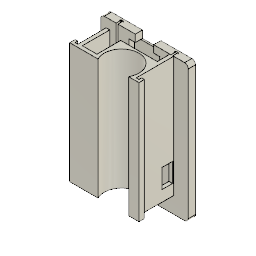
Battery Case v1 (Autodesk Fusion 360 design; units mm, degrees)
Autodesk Fusion 360 part; units mm, degrees
note: some values were not read from the file. Chosen so that the rebuilt part matches the saved one: which face or edge a step refers to; where a step starts. Set by a fixed rule: which sketch regions a step uses.
sketch "Bottom" plane through (0, 0, 0) normal (0, 1, 0) x (1, 0, 0) in component "Battery"
  line L0 (32.7362, 0) -> (32.7362, -7)
  line L1 (32.7362, -7) -> (12.7362, -7)
  line L2 (12.7362, -7) -> (12.7362, -20)
  line L3 (4.7362, 0) -> (4.7362, -20)
  line L4 (4.7362, -20) -> (12.7362, -20)
  line L5 (2.7362, 0) -> (2.7362, -20.5)
  line L6 (-0.2638, -22) -> (-0.2638, -19)
  line L7 (-0.2638, -19) -> (1.2362, -19)
  line L8 (1.2362, -19) -> (1.2362, -20.5)
  line L9 (1.2362, -20.5) -> (2.7362, -20.5)
  line L10 (37.7362, -22) -> (37.7362, -19)
  line L11 (37.7362, -19) -> (36.2362, -19)
  line L12 (36.2362, -19) -> (36.2362, -20.5)
  line L13 (36.2362, -20.5) -> (34.7362, -20.5)
  line L14 (-0.2638, -22) -> (15.3696, -22)
  line L15 (32.1028, -22) -> (37.7362, -22)
  line L16 (34.7362, 0) -> (34.7362, -20.5)
  line L17 (0, 0) -> (2.7362, 0) construction
  line L18 (4.2362, 0) -> (4.2362, 2.4992)
  line L19 (4.3455, 3) -> (4.8463, 2.4992)
  line L20 (3.2362, 2.4992) -> (3.2362, 0)
  line L21 (3.127, 3) -> (2.6261, 2.4992)
  line L22 (4.2362, 2.4992) -> (4.8463, 2.4992)
  line L23 (2.6261, 2.4992) -> (3.2362, 2.4992)
  line L24 (3.7361, 3) -> (3.7362, 0) construction
  line L25 (2.7362, 0) -> (4.7362, 0)
  line L26 (3.127, 3) -> (4.3455, 3)
  line L27 (32.6219, 2.4973) -> (33.232, 2.4983)
  line L28 (33.1209, 3) -> (32.6219, 2.4973)
  line L29 (33.1209, 3) -> (34.3394, 3)
  line L30 (33.7361, 3) -> (33.7362, 0) construction
  line L31 (34.232, 2.5) -> (34.8421, 2.501)
  line L32 (34.3394, 3) -> (34.8421, 2.501)
  line L33 (33.232, 2.4983) -> (33.2362, 0)
  line L34 (34.2362, 0) -> (34.232, 2.5)
  line L35 (32.7362, 0) -> (34.7362, 0)
  line L36 (15.3696, -22) -> (32.1028, -22) construction
  line L37 (23.7362, -22) -> (23.7362, -8) construction
  arc A0 (32.1028, -22) -> (15.3696, -22) centre (23.7362, -17.5) ccw
  dimension "d8" = 32
  dimension "d43" = 0
  dimension "d44" = 0
  dimension "d45" = 0
  dimension "d46" = 0
  dimension "d65" = 1.5
  dimension "d66" = 1.5
  dimension "d68" = 1.5
  dimension "d69" = 1.5
  dimension "d70" = 3
  dimension "d71" = 3
  dimension "d72" = 15.6334
  dimension "d73" = 5.6334
  dimension "d74" = 20.5
  dimension "d75" = 20
  dimension "d76" = 8
  dimension "d77" = 1.5
  dimension "d79" = 20
  dimension "d80" = 13
  dimension "d81" = 7
  dimension "d82" = 2
  dimension "d83" = 20.5
  dimension "d84" = 1.5
  dimension "d85" = 2.7362
  dimension "d94" = 1
  dimension "d98" = 0.6101
  dimension "d99" = 0.7083
  dimension "d100" = 1.2185
  dimension "d101" = 0.5
  dimension "d102" = 0.6101
  dimension "d103" = 0.7083
  dimension "d105" = 2
  dimension "d106" = 3
  dimension "d107" = 1
  dimension "d108" = 0.6101
  dimension "d109" = 0.7083
  dimension "d110" = 1.2185
  dimension "d112" = 0.6101
  dimension "d113" = 0.7083
  dimension "d116" = 0.5
  dimension "d117" = 3
  dimension "d118" = 2.5
  dimension "d132" = 19
  measures "d8" distance of L16.start L5.start
  measures "d65" distance of L6.end L7.end
  measures "d66" distance of L7.end L8.end
  measures "d68" distance of L11.end L12.end
  measures "d69" distance of L10.end L11.end
  measures "d70" distance of L6.start L6.end
  measures "d71" distance of L10.start L10.end
  measures "d72" distance of L14.end L6.start
  measures "d73" distance of L15.start L10.start
  measures "d74" distance of L5.start L5.end
  measures "d75" distance of L3.start L3.end
  measures "d76" distance of L3.end L2.end
  measures "d77" distance of L8.end L5.end
  measures "d79" distance of L0.end L1.end
  measures "d80" distance of L1.end L2.end
  measures "d81" distance of L0.start L0.end
  measures "d82" distance of L16.start L0.start
  measures "d83" distance of L16.start L13.end
  measures "d84" distance of L12.end L13.end
  measures "d85" distance of L5.start L17.start
  measures "d94" distance of L20.end L18.start
  measures "d98" distance of L19.end L18.end
  measures "d99" distance of L19.end L19.start
  measures "d100" distance of L21.start L19.start
  measures "d101" distance of L5.start L20
  measures "d102" distance of L21.end L20.start
  measures "d103" distance of L21.end L21.start
  measures "d105" distance of L3.start L5.start
  measures "d106" distance of L25 L26
  measures "d107" distance of L33.end L34.start
  measures "d108" distance of L31.start L31.end
  measures "d109" distance of L31.end L29.end
  measures "d110" distance of L28.start L29.end
  measures "d112" distance of L27.start L27.end
  measures "d113" distance of L27.start L28.start
  measures "d116" distance of L0.start L33
  measures "d117" distance of L29 L35
  measures "d118" distance of L31.start L34.start
  measures "d132" diameter of A0
extrude "Extrude1" add sketch "Bottom" along normal blind 66 contours L0 L1 L2 L3 L4 L5 L6 L7 L8 L9 L10 L11 L12 L13 L14 L15 L16 L25 L35 A0 makes body 1 in component "Battery"
sketch "Side" plane through (2.7362, 0, 0) normal (-1, 0, 0) x (0, 0, 1) in component "Battery"
  line L0 (0, 0) -> (20.5, 0)
  line L1 (20.5, 66) -> (0, 66)
  line L2 (0, 66) -> (5, 66)
  line L3 (5, 66) -> (5, 56)
  line L4 (5, 56) -> (0, 56)
  line L5 (0, 0) -> (5, 0)
  line L6 (5, 0) -> (5, 10)
  line L7 (5, 10) -> (0, 10)
  line L8 (20.5, 0) -> (20.5, 66)
  line L9 (0, 66) -> (0, 0)
  dimension "d86" = 10
  dimension "d87" = 5
  dimension "d88" = 10
  dimension "d89" = 5
  measures "d86" distance of L5.end L6.end
  measures "d87" distance of L6.end L7.end
  measures "d88" distance of L2.end L3.end
  measures "d89" distance of L3.end L4.end
extrude "Extrude2" cut sketch "Side" against normal blind 2 contours L0 L5 L6 L7 L9 | L1 L2 L3 L4 L9 bodies 1 in component "Battery"
sketch "Right Side" plane through (34.7362, 0, 0) normal (1, 0, 0) x (0, 0, -1) in component "Battery"
  line L0 (-22, 0) -> (0, 0)
  line L1 (0, 0) -> (0, 66)
  line L2 (0, 66) -> (-22, 66)
  line L3 (-22, 66) -> (-22, 0)
  line L4 (-0.6, 6) -> (-0.6, 16.5)
  line L5 (-6.4, 16.5) -> (-6.4, 6)
  line L6 (-0.6, 16.5) -> (-6.4, 16.5)
  line L7 (-6.4, 16.5) -> (-0.6, 16.5)
  line L8 (-0.6, 16.5) -> (-0.6, 6)
  line L9 (-0.6, 6) -> (-6.4, 6)
  line L10 (-6.4, 6) -> (-6.4, 16.5)
  line L11 (-20.5, 0) -> (0, 0)
  line L12 (0, 66) -> (-20.5, 66)
  line L13 (-20.5, 66) -> (-20.5, 0)
  line L14 (-0.6, 6) -> (0, 6) construction
  line L15 (0, 0) -> (0, 66)
  dimension "d14" = 10.5
  dimension "d90" = 6
  dimension "d91" = 0.6
  dimension "d92" = 5.8
  measures "d14" distance of L5.start L5.end
  measures "d90" distance of L0.end L14.end
  measures "d91" distance of L4.start L14.end
  measures "d92" distance of L4.start L5.end
extrude "Extrude3" cut sketch "Right Side" against normal blind 3 contours L4 L5 L6 L7 L8 L9 L10 bodies 1 in component "Battery"
extrude "Extrude9" add sketch "Bottom" against normal blind 40 from surface at 56 contours L18 L19 L20 L21 L22 L23 L25 L26 bodies 1 in component "Battery"
extrude "Extrude11" add sketch "Bottom" against normal blind 50 from surface at 66 contours L27 L28 L29 L31 L32 L33 L34 L35 bodies 1 in component "Battery"
extrude "Extrude10" cut sketch "Bottom" along normal blind 20 from surface at 26 contours L18 L19 L20 L21 L22 L23 L25 L26 bodies 1 in component "Battery"
extrude "Extrude12" cut sketch "Bottom" against normal blind 30 from surface at 56 contours L27 L28 L29 L31 L32 L33 L34 L35 bodies 1 in component "Battery"
sketch "Bottom (2)" plane through (0, 0, 0) normal (0, 1, 0) x (1, 0, 0) in component "Charger"
  line L0 (24, -2) -> (24, -73)
  line L1 (22, -75) -> (-22, -75)
  line L2 (-24, -73) -> (-24, -2)
  arc A0 (-22, 0) -> (-24, -2) centre (-22, -2) ccw
  arc A1 (24, -2) -> (22, 0) centre (22, -2) ccw
  arc A2 (22, -75) -> (24, -73) centre (22, -73) ccw
  arc A3 (-24, -73) -> (-22, -75) centre (-22, -73) ccw
  line L3 (5, 0) -> (5, -4)
  line L4 (5, -4) -> (-5, -4)
  line L5 (-5, -4) -> (-5, 0)
  line L6 (15.5, 0) -> (15.5, -50)
  line L7 (-15.5, -50) -> (-15.5, 0)
  line L8 (-15.5, 0) -> (-14.5, 0)
  line L9 (-14.5, 0) -> (-14.5, -50)
  line L10 (-14.5, -50) -> (-15.5, -50)
  line L11 (-15.5, -50) -> (-15.5, 0)
  line L12 (15.5, 0) -> (14.5, 0)
  line L13 (14.5, 0) -> (14.5, -50)
  line L14 (14.5, -50) -> (15.5, -50)
  line L15 (15.5, -50) -> (15.5, 0)
  line L16 (8.35, -4) -> (8.35, -30)
  line L17 (8.35, -30) -> (-8.45, -30)
  line L18 (-8.45, -4) -> (-8.45, -30)
  line L19 (-5, -4) -> (-8.45, -4)
  line L20 (5, -4) -> (8.35, -4)
  line L21 (0, -75) -> (0, 0) construction
  line L22 (22, 0) -> (5, 0)
  line L23 (-5, 0) -> (-22, 0)
  point P0 (-24, 0)
  point P1 (24, 0)
  point P2 (24, -75)
  dimension "d33" = 75
  dimension "d34" = 2
  dimension "d35" = 2
  dimension "d100_1" = 31
  dimension "d102_1" = 1
  dimension "d103_1" = 50
  dimension "d104" = 1
  dimension "d105_1" = 50
  dimension "d133" = 48
  dimension "d134" = 8.5
  dimension "d135" = 8.5
  dimension "d136" = 16.8
  dimension "d137" = 26
  dimension "d138" = 3.45
  dimension "d139" = 4
  dimension "d140" = 4
  dimension "d141" = 17
  dimension "d142" = 17
  measures "d33" distance of P1 P2
  measures "d34" radius of A0
  measures "d35" radius of A1
  measures "d100_1" distance of L7.end L6.start
  measures "d102_1" distance of L7.end L8.end
  measures "d103_1" distance of L7.end L7.start
  measures "d104" distance of L6.start L12.end
  measures "d105_1" distance of L6.start L6.end
  measures "d133" distance of L0 L2
  measures "d134" distance of L0 L6.end
  measures "d135" distance of L2 L7.start
  measures "d136" distance of L16.end L17.end
  measures "d137" distance of L17.end L18.start
  measures "d138" distance of L4.end L18.start
  measures "d139" distance of L5.end L4.end
  measures "d140" distance of L3.start L3.end
  measures "d141" distance of A0.start L5.end
  measures "d142" distance of A1.end L3.start
extrude "Extrude23" add sketch "Bottom (2)" along normal blind 4 separate body makes body 2 in component "Charger"
extrude "Extrude24" cut sketch "Bottom (2)" against normal blind 3 from surface at 4 contours L6 L12 L13 L14 L15 L22 | L4 L16 L17 L18 L19 L20 | L7 L8 L9 L10 L11 L23 bodies 2 in component "Charger"
sketch "Side (2)" plane through (0, 0, 0) normal (0, 0, -1) x (-1, 0, 0) in component "Charger"
  line L0 (-79.5, 0) -> (-78.5, 0)
  line L1 (16, 1.5) -> (14, 1.5)
  line L2 (14.5, 1) -> (14, 1.5)
  line L3 (15.5, 1) -> (16, 1.5)
  line L4 (14.5, 1) -> (14.5, 4)
  line L5 (14.5, 4) -> (5, 4)
  line L6 (5, 4) -> (5, 0)
  line L7 (5, 0) -> (22, 0)
  line L8 (22, 0) -> (22, 4)
  line L9 (22, 4) -> (15.5, 4)
  line L10 (15.5, 4) -> (15.5, 1)
  line L11 (15.5, 1) -> (14.5, 1)
extrude "Extrude25" cut sketch "Side (2)" against normal blind 50 contours L1 L3 L10 | L1 L4 L10 L11 | L1 L2 L4 bodies 2 in component "Charger"
mirror "Mirror1" about plane through (0, 0, 0) normal (1, 0, 0) of "Extrude25" in component "Charger"
component "Battery" placed x (1, 0, 0) y (0, 0, 1) z (0, -1, 0) at (-15, 21.8702, 0.3889)
component "Charger" placed x (1, 0, 0) y (0, -1, 0) z (0, 0, -1) at (3.7362, 25.8702, 66.3889)
equation "d65 = d66"
equation "d66 = d70 / 2"
equation "d68 = d66"
equation "d69 = d65"
equation "d71 = d70"
equation "d77 = d66"
equation "d84 = d68"
equation "d87 = d86 / 2"
equation "d88 = d86"
equation "d89 = d87"
equation "d102 = d98"
equation "d103 = d99"
equation "d112 = d98"
equation "d113 = d99"
equation "d132 = d_ext_cane"
equation "d_ext_cane = 19 mm" comment "Exterior diameter of the case"
equation "d35 = d34"
equation "d102_1 = d104"
equation "d103_1 = d105_1"
equation "d135 = d134"
equation "d140 = d139"
equation "d142 = d141"
named bodies: "Battery", "Charger"
